Regalplatte_Badezimmer_v1 (Autodesk Fusion 360 design; units mm, degrees)
Autodesk Fusion 360 part; units mm, degrees
sketch "Skizze1" plane through (0, 0, 0) normal (0, 1, 0) x (1, 0, 0)
  line L0 (5, 0) -> (35, 0)
  line L1 (40, -5) -> (40, -45)
  line L2 (35, -50) -> (5, -50)
  line L3 (0, -45) -> (0, -5)
  arc A0 (5, 0) -> (0, -5) centre (5, -5) ccw
  arc A1 (40, -5) -> (35, 0) centre (35, -5) ccw
  arc A2 (35, -50) -> (40, -45) centre (35, -45) ccw
  arc A3 (0, -45) -> (5, -50) centre (5, -45) ccw
  circle A4 centre (8, -42) radius 2
  circle A5 centre (32, -42) radius 2
  circle A6 centre (8, -8) radius 2
  circle A7 centre (32, -8) radius 2
  point P0 (0, -50)
  dimension "d1" = 50
  dimension "d2" = 5
  dimension "d3" = 5
  dimension "d4" = 5
  dimension "d5" = 5
  dimension "d6" = 40
  dimension "d8" = 4
  dimension "d9" = 4
  dimension "d10" = 8
  dimension "d11" = 8
  dimension "d12" = 8
  dimension "d13" = 8
  dimension "d19" = 4
  dimension "d20" = 4
  dimension "d21" = 8
  dimension "d22" = 8
  constraint horizontal L0
  constraint vertical L1
  constraint horizontal L2
  constraint vertical L3
  constraint coincident origin L3
  constraint coincident origin L0
  constraint tangent L3 A0
  constraint tangent L0 A0
  constraint tangent L0 A1
  constraint tangent L1 A1
  constraint tangent L1 A2
  constraint tangent L2 A2
  constraint coincident P0 L3
  constraint coincident P0 L2
  constraint tangent L3 A3
  constraint tangent L2 A3
  measures "d1" distance of origin P0
  measures "d2" radius of A0
  measures "d3" radius of A1
  measures "d4" radius of A2
  measures "d5" radius of A3
  measures "d6" distance of L1 L3
  measures "d8" diameter of A4
  measures "d9" diameter of A5
  measures "d10" distance of L3 A4.centre
  measures "d11" distance of L1 A5.centre
  measures "d12" distance of L2 A5.centre
  measures "d13" distance of L2 A4.centre
  measures "d19" diameter of A6
  measures "d20" diameter of A7
  measures "d21" distance of L0 A6.centre
  measures "d22" distance of L0 A7.centre
extrude "Extrusion1" add sketch "Skizze1" along normal blind 6
chamfer "Fase1" distance 3 angle 45 2 edges at (30.1353, 6, 41.2768) (6.1353, 6, 41.2768)
chamfer "Fase1" distance 3 angle 45 2 edges at (30.1353, 6, 7.2768) (6.1353, 6, 7.2768)
fillet "Abrundung1" radius 0.8 18 faces at (40, 2, 18.3333) (36.6353, 4, 0.275) (15, 2, 0) (2.7089, 4, 0.5558) (0, 2, 31.6667) (2.7089, 4, 49.4442) (25, 2, 50) (38.0908, 4, 48.9303) (17.0391, 6, 20.6364) (9.9975, 2, 42.0997) (32.9643, 5.3333, 12.2247) (10.1667, 5.3333, 38.2472) (34.1667, 5.3333, 38.2472) (9.9975, 2, 8.0997) (33.9975, 2, 42.0997) (33.9975, 2, 8.0997) (16.4157, 0, 19.8546) (10.1667, 5.3333, 11.7528)
equation "d2 = d3"
equation "d4 = d3"
equation "d5 = d3"
equation "d7 = 4 mm"
equation "d8 = d7"
equation "d9 = d7"
equation "d10 = d12"
equation "d11 = d12"
equation "d13 = d12"
equation "d19 = d7"
equation "d20 = d7"
equation "d22 = d21"
